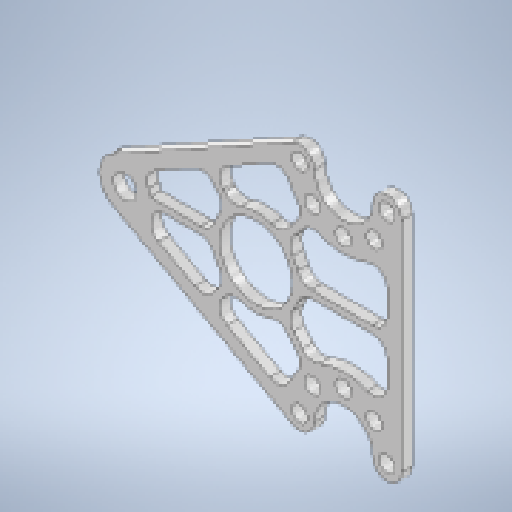
# Autodesk Inventor part: hiza
Saved by Autodesk Inventor 2025.1 (Build 291241000, 241)
## iProperties
Created: 2024-09-02
Part Number: hiza
Material: アルミニウム 2014-T4
Document SubType Name: Modeling
Designer: right
Density: 2.8 g/cm^3
Appearance: サテン
Mass: 1.97999 g
Surface Area: 16.4748 cm^2
Volume: 0.707138 cm^3
Author: right
Autodesk Inventor part; units mm, degrees
ref_plane "YZ Plane" through (0, 0, 0) normal (1, 0, 0) x (0, 1, 0)
ref_plane "XZ Plane" through (0, 0, 0) normal (0, 1, 0) x (-1, 0, 0)
ref_plane "XY Plane" through (0, 0, 0) normal (0, 0, 1) x (1, 0, 0)
sketch "スケッチ1" plane through (0, 0, 0) normal (0, 0, 1) x (1, 0, 0)
  line L0 (5.096, 0) -> (-5.096, 0) construction
  circle A0 centre (20, 15) radius 4
  circle A1 centre (20, 15) radius 8
  circle A2 centre (20, 15) radius 6 construction
  circle A3 centre (20, 21) radius 1.1
  circle A4 centre (15.7574, 19.2426) radius 1.1
  circle A5 centre (14, 15) radius 1.1
  circle A6 centre (15.7574, 10.7574) radius 1.1
  circle A7 centre (20, 9) radius 1.1
  circle A8 centre (24.2426, 10.7574) radius 1.1
  circle A9 centre (26, 15) radius 1.1
  circle A10 centre (24.2426, 19.2426) radius 1.1
  circle A11 centre (-10, 0) radius 1.6
  circle A12 centre (20, -15) radius 4
  circle A13 centre (20, -15) radius 8
  circle A14 centre (20, -15) radius 6 construction
  circle A15 centre (20, -21) radius 1.1
  circle A16 centre (15.7574, -19.2426) radius 1.1
  circle A17 centre (14, -15) radius 1.1
  circle A18 centre (15.7574, -10.7574) radius 1.1
  circle A19 centre (20, -9) radius 1.1
  circle A20 centre (24.2426, -10.7574) radius 1.1
  circle A21 centre (26, -15) radius 1.1
  circle A22 centre (24.2426, -19.2426) radius 1.1
  circle A23 centre (-10, 0) radius 1.6
  circle A24 centre (-10, 0) radius 3.5
  circle A25 centre (-10, 0) radius 3.5
  line L1 (-11.6951, 3.0621) -> (13.0314, 16.7498)
  line L2 (28, 15) -> (28, -15)
  circle A26 centre (14, 15) radius 2
  circle A27 centre (26, 15) radius 2
  line L3 (-11.6951, -3.0621) -> (13.0314, -16.7498)
  circle A28 centre (14, -15) radius 2
  circle A29 centre (26, -15) radius 2
  line L4 (-13.5, 0) -> (-13.5, 0)
  point P0 (0, 0)
  point P1 (0, 0)
  point P2 (12.0954, 16.2317)
  point P3 (12.0954, -16.2317)
  point P4 (28, -15)
  point P5 (28, 15)
  point P6 (24, 15)
  point P7 (16, 15)
  point P8 (-11.6951, -3.0621)
  point P9 (12.0954, -16.2317)
  point P10 (12, -15)
  point P11 (16, -15)
  point P12 (24, -15)
  dimension "d2" = 12
  dimension "d0" = 8
  dimension "d1" = 16
  dimension "d3" = 2.2
  dimension "d6" = 360
  dimension "d9" = 3.2
  dimension "d10" = 30
  dimension "d11" = 15
  dimension "d12" = 20
  dimension "d13" = 7
  constraints: 24 centre point, 17 symmetric about line, 10 end point, 9 coincident, 4 point on circle, 4 tangent, 3 horizontal, 3 vertical alignment, 2 midpoint, 2 point on line, 2 vertical, 1 line through centre, 47 other
  measures "d0" diameter of A0
  measures "d1" diameter of A1
  measures "d3" diameter of A3
  measures "d9" diameter of A11
  measures "d10" horizontal distance of A0.centre A11.centre
  measures "d11" vertical distance of A11.centre A0.centre
  measures "d12" horizontal distance of point (0, 0) A0.centre
  measures "d13" diameter of A24
extrude "押し出し1" add sketch "スケッチ1" along normal blind 1.5 contours A27 A1 A26 A0 | A27 | A26 | L2 A13 L3 A24 L1 A1 | A26 A1 L1 | A29 A12 A28 A13 | A29 | A24 | A28 L3 A13 | A28
sketch "スケッチ3" plane through (0, 0, 0) normal (0, 0, -1) x (-1, 0, 0)
  arc A0 (-24, 15) -> (-28, 15) centre (-26, 15) ccw projected
  line L0 (-28, -15) -> (-28, 15) projected
  arc A1 (-28, -15) -> (-24, -15) centre (-26, -15) ccw projected
  arc A2 (-16, -15) -> (-24, -15) centre (-20, -15) ccw projected
  arc A3 (-16, -15) -> (-13.0314, -16.7498) centre (-14, -15) ccw projected
  line L1 (11.6951, -3.0621) -> (-13.0314, -16.7498) projected
  arc A4 (11.6951, -3.0621) -> (11.6951, 3.0621) centre (10, 0) ccw projected
  line L2 (-13.0314, 16.7498) -> (11.6951, 3.0621) projected
  arc A5 (-13.0314, 16.7498) -> (-16, 15) centre (-14, 15) ccw projected
  arc A6 (-24, 15) -> (-16, 15) centre (-20, 15) ccw projected
  circle A7 centre (-14, 15) radius 1.1 projected
  circle A8 centre (-26, 15) radius 1.1 projected
  circle A9 centre (-14, -15) radius 1.1 projected
  circle A10 centre (-26, -15) radius 1.1 projected
  circle A11 centre (-24.2426, -10.7574) radius 1.1 projected
  circle A12 centre (-20, -9) radius 1.1 projected
  circle A13 centre (-15.7574, -10.7574) radius 1.1 projected
  circle A14 centre (10, 0) radius 1.6 projected
  circle A15 centre (-24.2426, 10.7574) radius 1.1 projected
  circle A16 centre (-20, 9) radius 1.1 projected
  circle A17 centre (-15.7574, 10.7574) radius 1.1 projected
  circle A18 centre (-20, 15) radius 8
  circle A19 centre (-20, -15) radius 8
  circle A20 centre (10, 0) radius 3.5
  arc A21 (10.7265, -1.3123) -> (10.7265, 1.3123) centre (10, 0) ccw
  line L3 (10.7265, -1.3123) -> (-14, -15)
  arc A22 (-14, -15) -> (-26, -15) centre (-20, -15) ccw
  line L4 (-26, -15) -> (-26, 15)
  arc A23 (-26, 15) -> (-14, 15) centre (-20, 15) ccw
  line L5 (-14, 15) -> (10.7265, 1.3123)
  line L6 (-26, 0) -> (10, 0) construction
  circle A24 centre (-8, 0) radius 5
  circle A25 centre (-8, 0) radius 6
  line L7 (-26, -0.5) -> (10, -0.5)
  line L8 (10, -0.5) -> (10, 0.5)
  line L9 (10, 0.5) -> (-26, 0.5)
  line L10 (-26, 0.5) -> (-26, -0.5)
  line L11 (-26, -0.5) -> (10, 0.5) construction
  line L12 (10, -0.5) -> (-26, 0.5) construction
  line L13 (4.3904, 14.6877) -> (-19.6096, -15.3123)
  line L14 (-19.6096, -15.3123) -> (-20.3904, -14.6877)
  line L15 (-20.3904, -14.6877) -> (3.6096, 15.3123)
  line L16 (3.6096, 15.3123) -> (4.3904, 14.6877)
  line L17 (4.3904, 14.6877) -> (-20.3904, -14.6877) construction
  line L18 (-19.6096, -15.3123) -> (3.6096, 15.3123) construction
  line L19 (4.3904, -14.6877) -> (-19.6096, 15.3123)
  line L20 (-20.3904, 14.6877) -> (3.6096, -15.3123)
  point P0 (0, 0)
  point P1 (-3.8744, -4.3566)
  point P2 (-1.0809, -7.8485)
  point P3 (7.9598, -2.8439)
  point P4 (6.5359, -0.5)
  point P5 (-2.0209, -0.5)
  point P6 (-14.6218, 9.0776)
  point P7 (-11.3447, 4.9813)
  point P8 (-4.6553, 4.9813)
  point P9 (-1.9685, 8.3398)
  point P10 (-12.0715, 13.9325)
  point P11 (-1.0809, 7.8485)
  point P12 (-3.8744, 4.3566)
  point P13 (-2.0209, 0.5)
  point P14 (6.5359, 0.5)
  point P15 (7.9598, 2.8439)
  point P16 (-1.9685, -8.3398)
  point P17 (-4.6553, -4.9813)
  point P18 (-11.3447, -4.9813)
  point P19 (-14.6218, -9.0776)
  point P20 (-12.0715, -13.9325)
  point P21 (-15.4026, -8.4529)
  point P22 (-12.1256, -4.3566)
  point P23 (-13.9791, -0.5)
  point P24 (-26, -9.7085)
  point P25 (-12.1256, 4.3566)
  point P26 (-15.4026, 8.4529)
  point P27 (-26, 9.7085)
  point P28 (-13.9791, 0.5)
  dimension "d27" = 2
  dimension "d28" = 10
  dimension "d29" = 12
  dimension "d30" = 1
  dimension "d31" = 1
  constraints: 36 end point, 7 midpoint, 6 point on circle, 5 centre point, 5 coincident, 5 parallel, 4 symmetric about line, 3 perpendicular, 14 other
  measures "d27" distance between parallel lines of L2 L5
  measures "d28" diameter of A24
  measures "d29" diameter of A25
  measures "d30" distance of L8.end L7.end
  measures "d31" distance of L13.end L14.end
extrude "押し出し3" cut sketch "スケッチ3" against normal through all contours A18 L20 A25 L9 L4 | L4 L7 A25 L15 A19 | L15 A25 L19 A18 L5 | L13 A25 L20 L3 A19 | L5 A20 L9 A25 L13 | L20 L9 A24 | A24 L19 L15 L9 L20 | L9 L20 L15 L7 A24 | L15 L7 L20 L13 A24 | A24 L7 L15 | L19 A25 L7 A20 L3 | L15 L19 A24 | A24 L13 L9 L19 L15 | L9 L15 L20 | L13 L20 A24 | L15 L20 L7 | L20 L13 L7 L19 A24 | A24 L9 L13 | L19 L9 L15 | L9 L19 L13 L7 L20 L15 | L20 L7 L13 | L19 L7 A24 | A24 L7 L19 L13 L9 | L13 L19 L9 | L13 L19 L7
fillet "フィレット2" radius 2 29 edges at (26, -0.5, 0.75) (26, 0.5, 0.75) (13.9791, -0.5, 0.75) (13.9791, 0.5, 0.75) (26, -9.7085, 0.75) (15.4026, -8.4529, 0.75) (12.1256, -4.3566, 0.75) (11.3447, -4.9813, 0.75) (14.6218, -9.0776, 0.75) (12.0715, -13.9325, 0.75) (1.9685, -8.3398, 0.75) (1.0809, -7.8485, 0.75) (4.6553, -4.9813, 0.75) (3.8744, -4.3566, 0.75) (2.0209, -0.5, 0.75) (2.0209, 0.5, 0.75) (-6.5359, -0.5, 0.75) (-7.9598, -2.8439, 0.75) (-7.9598, 2.8439, 0.75) (1.0809, 7.8485, 0.75) (3.8744, 4.3566, 0.75) (4.6553, 4.9813, 0.75) (1.9685, 8.3398, 0.75) (11.3447, 4.9813, 0.75) (14.6218, 9.0776, 0.75) (15.4026, 8.4529, 0.75) (12.1256, 4.3566, 0.75) (26, 9.7085, 0.75) (12.0715, 13.9325, 0.75)
